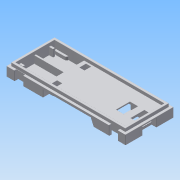
# Autodesk Inventor part: D2MG основание
Saved by Autodesk Inventor 2015 SP1 (Build 190203100, 203)
## iProperties
Created: 2017-11-06
Part Number: D2MG основание
Material: Типовые
Document SubType Name: Modeling
Designer: Влад
Density: 1 g/cm^3
Appearance: Белый пластик
Author: Влад
Autodesk Inventor part; units mm, degrees
ref_plane "YZ Plane" through (0, 0, 0) normal (1, 0, 0) x (0, 1, 0)
sketch "Эскиз1" plane through (0, 0, 0) normal (0, 0, 1) x (1, 0, 0)
  line L0 (-45.1, 18.15) -> (45.1, 18.15)
  line L1 (45.1, 18.15) -> (45.1, -18.15)
  line L2 (45.1, -18.15) -> (-45.1, -18.15)
  line L3 (-45.1, -18.15) -> (-45.1, 18.15)
  line L4 (-45.1, 18.15) -> (45.1, -18.15) construction
  line L5 (45.1, 18.15) -> (-45.1, -18.15) construction
  point P0 (0, 0)
  point P1 (0, 0)
  dimension "d0" = 90.2
  dimension "d1" = 36.3
  constraints: 12 end point, 2 parallel, 1 coincident, 1 horizontal, 1 midpoint, 1 perpendicular
  measures "d0" distance of L1.end L2.end
  measures "d1" distance of L0.end L1.end
extrude "Выдавливание1" add sketch "Эскиз1" along normal blind 2
sketch "Эскиз2" plane through (0, 0, 2) normal (0, 0, 1) x (1, 0, 0)
  line L0 (-43.25, 16.45) -> (43.25, 16.45)
  line L1 (43.25, 16.45) -> (43.25, -16.45)
  line L2 (43.25, -16.45) -> (-43.25, -16.45)
  line L3 (-43.25, -16.45) -> (-43.25, 16.45)
  line L4 (45.1, -18.15) -> (45.1, 18.15) projected
  line L5 (-45.1, 18.15) -> (-45.1, -18.15) projected
  line L6 (45.1, 18.15) -> (-45.1, 18.15) projected
  line L7 (-45.1, -18.15) -> (45.1, -18.15) projected
  line L8 (-41.55, 14.75) -> (41.55, 14.75)
  line L9 (41.55, 14.75) -> (41.55, -14.75)
  line L10 (41.55, -14.75) -> (-41.55, -14.75)
  line L11 (-41.55, -14.75) -> (-41.55, 14.75)
  point P0 (0, 0)
  dimension "d102" = 14.15
  dimension "d4" = 1.85
  dimension "d5" = 1.85
  dimension "d6" = 1.7
  dimension "d7" = 1.7
  dimension "d8" = 1.7
  dimension "d9" = 1.7
  dimension "d10" = 1.7
  dimension "d11" = 1.7
  constraints: 16 end point, 4 parallel, 2 horizontal, 2 perpendicular
  measures "d4" distance between parallel lines of L4 L1
  measures "d5" distance between parallel lines of L5 L3
  measures "d6" distance between parallel lines of L6 L0
  measures "d7" distance between parallel lines of L7 L2
  measures "d8" distance between parallel lines of L0 L8
  measures "d9" distance between parallel lines of L2 L10
  measures "d10" distance between parallel lines of L1 L9
  measures "d11" distance between parallel lines of L3 L11
extrude "Выдавливание2" add sketch "Эскиз2" along normal blind 2.4 contours L0 L1 L2 L3
sketch "Эскиз3" plane through (0, 0, 0) normal (0, 0, -1) x (-1, 0, 0)
  line L0 (7.1, -5.25) -> (-45.1, -5.25)
  line L1 (-45.1, -5.25) -> (-45.1, 5.25)
  line L2 (-45.1, 5.25) -> (7.1, 5.25)
  line L3 (7.1, 5.25) -> (7.1, -5.25)
  line L4 (45.1, -18.15) -> (45.1, 18.15) projected
  line L5 (-45.1, 18.15) -> (-45.1, -18.15) projected
  line L6 (45.1, 18.15) -> (-45.1, 18.15) projected
  line L7 (-45.1, -18.15) -> (45.1, -18.15) projected
  point P0 (0, 0)
  point P1 (-45.1, 0)
  dimension "d14" = 10.5
  dimension "d15" = 38
  dimension "d66" = 12.9
  dimension "d67" = 12.9
  constraints: 8 end point, 2 midpoint, 2 parallel, 1 horizontal, 1 perpendicular
  measures "d14" distance of L0.end L1.end
  measures "d15" distance between parallel lines of L4 L3
  measures "d66" distance between parallel lines of L6 L2
  measures "d67" distance between parallel lines of L7 L0
extrude "Выдавливание3" cut sketch "Эскиз3" against normal blind 1.1 contours L0 L1 L2 L3
sketch "Эскиз4" plane through (0, 0, 0) normal (0, 0, -1) x (-1, 0, 0)
  line L0 (-45.1, 18.15) -> (45.1, 18.15) projected
  line L1 (45.1, -18.15) -> (17.4, -18.15)
  line L2 (17.4, -18.15) -> (17.4, 18.15)
  line L3 (17.4, 18.15) -> (45.1, 18.15)
  line L4 (45.1, 18.15) -> (45.1, -18.15)
  point P0 (0, 0)
  dimension "d18" = 27.7
  constraints: 8 end point, 2 parallel, 1 horizontal, 1 perpendicular, 1 point on line
  measures "d18" distance of L2.end L3.end
extrude "Выдавливание4" add sketch "Эскиз4" along normal blind 5.1
sketch "Эскиз5" plane through (0, 0, -5.1) normal (0, 0, -1) x (-1, 0, 0)
  line L0 (39.1, -18.15) -> (32.6, -18.15)
  line L1 (32.6, -18.15) -> (32.6, -16.65)
  line L2 (32.6, -16.65) -> (39.1, -16.65)
  line L3 (39.1, -16.65) -> (39.1, -18.15)
  line L4 (39.1, 16.65) -> (32.6, 16.65)
  line L5 (32.6, 16.65) -> (32.6, 18.15)
  line L6 (32.6, 18.15) -> (39.1, 18.15)
  line L7 (39.1, 18.15) -> (39.1, 16.65)
  line L8 (45.1, -18.15) -> (45.1, 18.15) projected
  line L9 (17.4, -18.15) -> (45.1, -18.15) projected
  line L10 (45.1, 18.15) -> (17.4, 18.15) projected
  point P0 (0, 0)
  point P1 (35.85, -18.15)
  point P2 (35.85, 18.15)
  dimension "d21" = 6.5
  dimension "d22" = 1.5
  dimension "d23" = 6.5
  dimension "d24" = 1.5
  dimension "d25" = 6
  dimension "d26" = 6
  constraints: 16 end point, 4 parallel, 3 point on line, 2 horizontal, 2 midpoint, 2 perpendicular
  measures "d21" distance of L1.end L2.end
  measures "d22" distance of L0.end L1.end
  measures "d23" distance of L5.end L6.end
  measures "d24" distance of L4.end L5.end
  measures "d25" distance between parallel lines of L8 L3
  measures "d26" distance between parallel lines of L8 L7
extrude "Выдавливание5" cut sketch "Эскиз5" against normal through all
sketch "Эскиз6" plane through (0, 0, -5.1) normal (0, 0, -1) x (-1, 0, 0)
  line L0 (39.1, -16.65) -> (32.6, -16.65)
  line L1 (32.6, -16.65) -> (32.6, -15.15)
  line L2 (32.6, -15.15) -> (39.1, -15.15)
  line L3 (39.1, -15.15) -> (39.1, -16.65)
  line L4 (39.1, 16.65) -> (32.6, 16.65)
  line L5 (32.6, 16.65) -> (32.6, 15.15)
  line L6 (32.6, 15.15) -> (39.1, 15.15)
  line L7 (39.1, 15.15) -> (39.1, 16.65)
  point P0 (0, 0)
  dimension "d29" = 1.5
  dimension "d30" = 1.5
  constraints: 16 end point, 4 parallel, 2 horizontal, 2 perpendicular, 1 point on line
  measures "d29" distance of L0.end L1.end
  measures "d30" distance of L5.end L4.end
extrude "Выдавливание6" cut sketch "Эскиз6" against normal blind 3
sketch "Эскиз8" plane through (45.1, 18.15, 2) normal (0, 1, 0) x (1, 0, 0)
  line L0 (-26.5, 2) -> (-24.3, 7.1)
  line L1 (0, 7.1) -> (0, 2)
  line L2 (0, 2) -> (-62.5, 2) projected
  line L3 (-62.5, 2) -> (-62.5, 7.1) projected
  line L4 (-6, 7.1) -> (-6, 2)
  line L5 (-12.5, 2) -> (-12.5, 7.1)
  line L6 (-24.3, 7.1) -> (-12.5, 7.1)
  line L7 (-6, 7.1) -> (0, 7.1)
  line L8 (0, 2) -> (-6, 2)
  line L9 (-12.5, 2) -> (-26.5, 2)
  dimension "d34" = 36
  dimension "d35" = 38.2
  dimension "d38" = 6
  dimension "d39" = 6.5
  constraints: 16 end point, 2 collinear, 2 horizontal, 2 perpendicular, 2 point on line, 1 parallel
  measures "d34" distance of L2.end L0.start
  measures "d35" distance from line of L3 L0.end
  measures "d38" distance between parallel lines of L1 L4
  measures "d39" distance between parallel lines of L4 L5
extrude "Выдавливание7" add sketch "Эскиз8" against normal blind 2
sketch "Эскиз9" plane through (0, 0, 2) normal (0, 0, 1) x (1, 0, 0)
  line L0 (32.6, 18.15) -> (39.1, 18.15)
  line L1 (39.1, 18.15) -> (39.1, 16.45)
  line L2 (39.1, 16.45) -> (32.6, 16.45)
  line L3 (32.6, 16.45) -> (32.6, 18.15)
  line L4 (45.1, 16.15) -> (45.1, 5.25) projected
  line L5 (32.6, 18.15) -> (39.1, 18.15) projected
  point P0 (0, 0)
  point P1 (35.85, 18.15)
  dimension "d42" = 6.5
  dimension "d43" = 1.7
  dimension "d44" = 6
  constraints: 8 end point, 2 midpoint, 2 parallel, 1 horizontal, 1 perpendicular
  measures "d42" distance of L1.end L2.end
  measures "d43" distance of L0.end L1.end
  measures "d44" distance between parallel lines of L4 L1
extrude "Выдавливание8" cut sketch "Эскиз9" against normal blind 2
sketch "Эскиз10" plane through (0, 0, 0) normal (0, 0, -1) x (-1, 0, 0)
  line L0 (-45.1, 5.25) -> (7.1, 5.25) projected
  line L1 (-45.1, -18.15) -> (-45.1, 18.15) projected
  line L2 (-25.6, 5.25) -> (-45.1, 5.25)
  line L3 (-45.1, 5.25) -> (-45.1, 16.45)
  line L4 (-45.1, 16.45) -> (-43.1, 16.45)
  line L5 (-25.6, 7.25) -> (-25.6, 5.25)
  line L6 (-25.6, 7.25) -> (-43.1, 7.25)
  line L7 (-43.1, 7.25) -> (-43.1, 16.45)
  point P0 (0, 0)
  dimension "d47" = 19.5
  dimension "d48" = 2
  constraints: 12 end point, 2 horizontal, 2 parallel, 2 point on line, 1 perpendicular, 1 vertical
  measures "d47" distance between parallel lines of L1 L5
  measures "d48" distance between parallel lines of L6 L0
extrude "Выдавливание9" add sketch "Эскиз10" along normal blind 5.1
sketch "Эскиз11" plane through (0, 0, 0) normal (0, 0, -1) x (-1, 0, 0)
  line L0 (-31.1, 14.95) -> (-40.6, 14.95)
  line L1 (-40.6, 14.95) -> (-40.6, 16.45)
  line L2 (-40.6, 16.45) -> (-31.1, 16.45)
  line L3 (-31.1, 16.45) -> (-31.1, 14.95)
  line L4 (-39.1, 18.15) -> (-39.1, 16.45) projected
  line L5 (-32.6, 16.45) -> (-32.6, 18.15) projected
  line L6 (-43.25, 16.45) -> (43.25, 16.45) projected
  point P0 (0, 0)
  point P1 (-35.85, 16.45)
  dimension "d53" = 1.5
  dimension "d54" = 1.5
  dimension "d55" = 1.5
  constraints: 8 end point, 2 parallel, 1 horizontal, 1 midpoint, 1 perpendicular, 1 point on line
  measures "d53" distance between parallel lines of L4 L1
  measures "d54" distance between parallel lines of L5 L3
  measures "d55" distance between parallel lines of L2 L0
extrude "Выдавливание10" add sketch "Эскиз11" along normal blind 2
fillet "Сопряжение1" radius 1.5 2 edges at (31.1, 14.95, -1) (40.6, 14.95, -1)
sketch "Эскиз12" plane through (0, 0, 0) normal (0, 0, -1) x (-1, 0, 0)
  ellipse E0 centre (-22.9, 13.95) end of major axis (-24.5, 13.95) minor radius 1.2
  line L0 (7.1, 5.25) -> (7.1, -5.25) projected
  line L1 (-32.6, 18.15) -> (32.6, 18.15) projected
  point P0 (0, 0)
  dimension "d60" = 1.6
  dimension "d61" = 1.2
  dimension "d62" = 30
  dimension "d63" = 4.2
  constraints: 2 other
  measures "d62" distance from line of L0 point (-22.9, 13.95)
  measures "d63" distance from line of point (-22.9, 13.95) L1
extrude "Выдавливание11" add sketch "Эскиз12" along normal blind 3
mirror "Зеркальное отражение1" about plane through (0, 0, 0) normal (0, 1, 0) of "Выдавливание7", "Выдавливание8", "Выдавливание9", "Выдавливание10", "Сопряжение1", "Выдавливание11"
sketch "Эскиз15" plane through (45.1, -18.15, -5.1) normal (0, 0, -1) x (-1, 0, 0)
  line L0 (0, 23.4) -> (52.2, 23.4) projected
  line L1 (19.5, 12.9) -> (14.5, 12.9)
  line L2 (14.5, 12.9) -> (14.5, 23.4)
  line L3 (14.5, 23.4) -> (19.5, 23.4)
  line L4 (19.5, 23.4) -> (19.5, 12.9)
  line L5 (52.2, 12.9) -> (0, 12.9) projected
  line L6 (8.7, 12.9) -> (3.7, 12.9)
  line L7 (3.7, 12.9) -> (3.7, 23.4)
  line L8 (3.7, 23.4) -> (8.7, 23.4)
  line L9 (8.7, 23.4) -> (8.7, 12.9)
  point P0 (45.1, 18.15)
  dimension "d68" = 5
  dimension "d69" = 5
  dimension "d70" = 5.8
  constraints: 16 end point, 4 parallel, 3 point on line, 2 horizontal, 2 perpendicular
  measures "d68" distance of L2.end L3.end
  measures "d69" distance of L7.end L8.end
  measures "d70" distance between parallel lines of L9 L2
extrude "Выдавливание12" add sketch "Эскиз15" against normal blind 2 contours L0 L9 L5 L7 | L0 L4 L1 L2
sketch "Эскиз16" plane through (0, 0, 2) normal (0, 0, 1) x (1, 0, 0)
  line L0 (-7.1, -5.25) -> (45.1, -5.25) projected
  line L1 (-7.1, 5.25) -> (-7.1, -5.25) projected
  line L2 (45.1, 5.25) -> (-7.1, 5.25) projected
  line L3 (45.1, -5.25) -> (45.1, 5.25) projected
  line L4 (-7.1, -5.25) -> (45.1, -5.25) projected
  line L5 (36.1, 5.25) -> (42.1, 5.25)
  line L6 (42.1, 5.25) -> (42.1, -5.25)
  line L7 (42.1, -5.25) -> (36.1, -5.25)
  line L8 (36.1, -5.25) -> (36.1, 5.25)
  line L9 (45.1, 5.25) -> (-7.1, 5.25) projected
  line L10 (31.1, 5.25) -> (25.1, 5.25)
  line L11 (25.1, 5.25) -> (25.1, -5.25)
  line L12 (25.1, -5.25) -> (31.1, -5.25)
  line L13 (31.1, -5.25) -> (31.1, 5.25)
  point P0 (0, 0)
  dimension "d73" = 6
  dimension "d74" = 6
  dimension "d75" = 5
  dimension "d76" = 3
  constraints: 16 end point, 4 parallel, 4 point on line, 2 horizontal, 2 perpendicular
  measures "d73" distance of L6.end L7.end
  measures "d74" distance of L12.end L11.end
  measures "d75" distance between parallel lines of L8 L13
  measures "d76" distance between parallel lines of L3 L6
extrude "Выдавливание13" cut sketch "Эскиз16" against normal blind 2 contours L11 L2 L13 L0 | L8 L2 L6 L0
ref_plane "РабПлоскость1" through (-17.4, 13.35, 0) normal (0, 1, 0) x (1, 0, 0)
sketch "Эскиз17" plane through (-17.4, 13.35, 0) normal (0, 1, 0) x (1, 0, 0)
  line L0 (0, 5.1) -> (3, 5.1)
  line L1 (3, 5.1) -> (3, 3.4)
  line L2 (3, 3.4) -> (1, 2.1002)
  line L3 (1, 2.1002) -> (1, 0)
  line L4 (1, 0) -> (0, 0)
  line L5 (0, 0) -> (36, 0) projected
  line L6 (0, 0) -> (0, 5.1)
  point P0 (17.4, 0)
  dimension "d80" = 3
  dimension "d81" = 1.7
  dimension "d82" = 1
  constraints: 12 end point, 2 perpendicular, 1 collinear, 1 horizontal, 1 parallel
  measures "d80" distance of L0.start L0.end
  measures "d81" distance of L0.end L1.end
  measures "d82" distance of L3.end L4.end
extrude "Выдавливание14" add sketch "Эскиз17" against normal blind 4.8
ref_plane "РабПлоскость2" through (-17.4, 11.95, 0) normal (0, 1, 0) x (1, 0, 0)
sketch "Эскиз18" plane through (-17.4, 11.95, 0) normal (0, 1, 0) x (1, 0, 0)
  line L0 (3, 3.4) -> (3, 2.4328)
  line L1 (3, 2.4328) -> (1, 1.7474)
  line L2 (1, 2.1002) -> (1, 0) projected
  line L3 (1, 1.7474) -> (1, 2.1002)
  line L4 (3, 3.4) -> (1, 2.1002)
  point P0 (17.4, 0)
  constraints: 8 end point, 1 collinear, 1 point on line, 1 vertical
extrude "Выдавливание15" add sketch "Эскиз18" against normal blind 2
sketch "Эскиз19" plane through (0, 0, 0) normal (0, 0, -1) x (-1, 0, 0)
  line L0 (16.4, 8.45) -> (12.6, 8.45)
  line L1 (12.6, 8.45) -> (12.6, 13.45)
  line L2 (12.6, 13.45) -> (16.4, 13.45)
  line L3 (16.4, 13.45) -> (16.4, 8.45)
  line L4 (16.4, 8.55) -> (16.4, 13.35) projected
  line L5 (17.4, 18.15) -> (-18.6, 18.15) projected
  point P0 (0, 0)
  point P1 (16.4, 10.95)
  dimension "d88" = 3.8
  dimension "d89" = 5
  dimension "d90" = 4.7
  constraints: 8 end point, 2 midpoint, 2 parallel, 1 horizontal, 1 perpendicular
  measures "d88" distance between parallel lines of L4 L1
  measures "d89" distance between parallel lines of L2 L0
  measures "d90" distance between parallel lines of L5 L2
extrude "Выдавливание16" cut sketch "Эскиз19" against normal blind 2.5
mirror "Зеркальное отражение3" about plane through (0, 0, 0) normal (0, 1, 0) of "Выдавливание14", "Выдавливание15", "Выдавливание16"
sketch "Эскиз20" plane through (0, 0, 4.4) normal (0, 0, 1) x (1, 0, 0)
  line L0 (-41.55, 14.75) -> (-19.35, 14.75)
  line L1 (-19.35, 14.75) -> (-19.35, -14.75)
  line L2 (-19.35, -14.75) -> (-41.55, -14.75)
  line L3 (-41.55, -14.75) -> (-41.55, 14.75)
  line L4 (-41.55, -14.75) -> (41.55, -14.75) projected
  point P0 (0, 0)
  point P1 (-30.45, -14.75)
  dimension "d93" = 22.2
  dimension "d94" = 29.5
  constraints: 8 end point, 2 parallel, 1 horizontal, 1 midpoint, 1 perpendicular, 1 point on line
  measures "d93" distance of L1.end L2.end
  measures "d94" distance between parallel lines of L2 L0
extrude "Выдавливание17" cut sketch "Эскиз20" against normal blind 8
sketch "Эскиз21" plane through (0, 0, -3.6) normal (0, 0, 1) x (1, 0, 0)
  line L0 (-41.55, 14.75) -> (-19.35, 14.75) projected
  line L1 (-41.55, -14.75) -> (-41.55, 14.75) projected
  line L2 (-19.35, -14.75) -> (-41.55, -14.75) projected
  line L3 (-19.35, 14.75) -> (-19.35, -14.75) projected
  line L4 (-41.55, 0.6) -> (-19.35, 0.6)
  line L5 (-19.35, -0.6) -> (-41.55, -0.6)
  line L6 (-41.55, 12.1) -> (-38.55, 12.1)
  line L7 (-38.55, 12.1) -> (-38.55, 10.6)
  line L8 (-38.55, 10.6) -> (-41.55, 10.6)
  line L9 (-41.55, 10.6) -> (-41.55, 12.1)
  line L10 (-41.55, -10.6) -> (-38.55, -10.6)
  line L11 (-38.55, -10.6) -> (-38.55, -12.1)
  line L12 (-38.55, -12.1) -> (-41.55, -12.1)
  line L13 (-41.55, -12.1) -> (-41.55, -10.6)
  point P0 (0, 0)
  dimension "d101" = 14.15
  dimension "d102" = 14.15
  dimension "d103" = 1.2
  dimension "d106" = 3
  dimension "d107" = 1.5
  dimension "d108" = 10
  dimension "d109" = 3
  dimension "d110" = 1.5
  dimension "d111" = 10
  constraints: 20 end point, 6 point on line, 5 parallel, 3 horizontal, 2 perpendicular
  measures "d101" distance between parallel lines of L0 L4
  measures "d102" distance between parallel lines of L2 L5
  measures "d103" distance between parallel lines of L5 L4
  measures "d106" distance of L7.end L8.end
  measures "d107" distance of L6.end L7.end
  measures "d108" distance between parallel lines of L4 L8
  measures "d109" distance of L11.end L12.end
  measures "d110" distance of L10.end L11.end
  measures "d111" distance between parallel lines of L5 L10
extrude "Выдавливание19" add sketch "Эскиз21" along normal blind 5.5 contours L6 L7 L8 L1 | L3 L5 L1 L4 | L10 L11 L12 L1
sketch "Эскиз22" plane through (0, 0, -3.6) normal (0, 0, 1) x (1, 0, 0)
  line L0 (-40.6, -13.25) -> (-31.1, -13.25)
  line L1 (-31.1, -13.25) -> (-31.1, -14.75)
  line L2 (-31.1, -14.75) -> (-40.6, -14.75)
  line L3 (-40.6, -14.75) -> (-40.6, -13.25)
  line L4 (-39.1, -15.15) -> (-39.1, -18.15) projected
  line L5 (-32.6, -16.65) -> (-32.6, -18.15) projected
  line L6 (-32.6, -18.15) -> (-32.6, -15.15) projected
  line L7 (-19.35, -14.75) -> (-41.55, -14.75) projected
  point P0 (0, 0)
  point P1 (-35.85, -14.75)
  dimension "d114" = 1.5
  dimension "d115" = 1.5
  dimension "d117" = 1.5
  constraints: 8 end point, 2 parallel, 1 horizontal, 1 midpoint, 1 perpendicular, 1 point on line
  measures "d114" distance of L0.end L1.end
  measures "d115" distance between parallel lines of L4 L3
  measures "d117" distance between parallel lines of L6 L1
extrude "Выдавливание20" add sketch "Эскиз22" along normal blind 2.5
fillet "Сопряжение2" radius 1.5 2 edges at (-31.1, -13.25, -2.35) (-40.6, -13.25, -2.35)
mirror "Зеркальное отражение4" about plane through (0, 0, 0) normal (0, 1, 0) of "Выдавливание20", "Сопряжение2"
fillet "Сопряжение3" radius 0.1 26 edges at (-38.55, 10.6, -0.85) (-38.55, 12.1, -0.85) (-38.55, 11.35, 1.9) (-40.05, 10.6, 1.9) (-40.05, 12.1, 1.9) (-38.55, -11.35, 1.9) (-40.05, -12.1, 1.9) (-38.55, -12.1, -0.85) (-38.55, -10.6, -0.85) (-40.05, -10.6, 1.9) (-40.1607, 13.6893, -1.1) (-40.6, 14.7499, -1.1) (-31.5393, 13.6893, -1.1) (-31.1, 14.7499, -1.1) (-35.85, 13.25, -1.1) (-40.6, -14.7499, -1.1) (-40.1607, -13.6893, -1.1) (-31.5393, -13.6893, -1.1) (-31.1, -14.7499, -1.1) (-35.85, -13.25, -1.1) (31.621, -15.2881, -2) (40.079, -15.2881, -2) (35.85, -14.95, -2) (31.621, 15.2881, -2) (40.079, 15.2881, -2) (35.85, 14.95, -2)
fillet "Сопряжение4" radius 0.2 22 edges at (-19.35, 0, 2) (0, -18.15, 2) (-42.1, -18.15, 2) (-45.1, 0, 2) (-42.1, 18.15, 2) (-39.1, 17.4, 2) (-32.6, 17.4, 2) (0, 18.15, 2) (32.6, 17.3, 2) (39.1, 17.3, 2) (42.1, 18.15, 2) (45.1, 0, 2) (42.1, -18.15, 2) (39.1, -17.3, 2) (32.6, -17.3, 2) (43.25, 0, 4.4) (0, 16.45, 4.4) (43.25, 16.45, 3.2) (-43.25, 16.45, 3.2) (-43.25, 0, 4.4) (-43.25, -16.45, 3.2) (0, -16.45, 4.4)
fillet "Сопряжение5" radius 0.3 37 edges at (-45.1, 0, -5.1) (-42.1, 18.15, -5.1) (-45.0414, 18.0914, 1.9414) (-45.1, 18.15, -1.65) (-32.5414, 18.0914, 1.9414) (-32.6, 18.15, -1.65) (-39.1586, 18.0914, 1.9414) (-39.1, 18.15, -1.65) (-17.4, 18.15, -2.55) (-25, 18.15, -5.1) (-17.4, 15.75, -5.1) (-17.4, 0, -5.1) (-14.4, 10.95, -5.1) (-15.9, 13.35, -5.1) (-14.4, 13.35, -4.25) (-17.4, -15.75, -5.1) (-15.9, -13.35, -5.1) (-14.4, -10.95, -5.1) (-15.9, -8.55, -5.1) (-14.4, -8.55, -4.25) (-14.4, -13.35, -4.25) (-14.4, 8.55, -4.25) (0.6, 18.15, 0) (19.7, 18.15, -2.55) (26.7, 18.15, -5.1) (32.5414, 18.0914, 1.9414) (32.6, 18.15, -1.65) (42.1, 18.15, -5.1) (39.1586, 18.0914, 1.9414) (39.1, 18.15, -1.65) (45.0414, 18.0914, 1.9414) (45.1, 18.15, -1.65) (45.1, 11.7, -5.1) (45.1, 5.25, -2) (45.1, -5.25, -2) (45.0414, -18.0914, 1.9414) (45.1, -18.15, -1.65)
fillet "Сопряжение6" radius 0.3 13 edges at (-45.0121, -18.15, -5.0121) (-41.95, -18.15, -5.1) (-45.0414, -18.0914, 1.9414) (-45.1, -18.15, -1.5) (-17.4879, -18.15, -5.0121) (-17.4, -18.15, -2.4) (-25.15, -18.15, -5.1) (-32.6, -18.0914, 1.9414) (-32.6, -17.3, 2) (-32.6, -18.15, -1.65) (-39.1, -18.0914, 1.9414) (-39.1, -17.3, 2) (-39.1, -18.15, -1.65)
fillet "Сопряжение7" radius 0.3 12 edges at (0.45, -18.15, 0) (19.7, -18.15, -2.55) (26.7, -18.15, -5.1) (32.5414, -18.0914, 1.9414) (32.6, -18.15, -1.65) (39.1586, -18.0914, 1.9414) (39.1, -18.15, -1.65) (45.0121, -18.0621, -5.1) (45.1, -11.7, -5.1) (45.0121, -5.3379, -5.1) (43.1, -5.25, -5.1) (41.95, -18.15, -5.1)
fillet "Сопряжение8" radius 0.2 11 edges at (25.6, 0, -5.1) (41.4, -0.15, -5.1) (45.0121, 5.3379, -5.0121) (43.1, 5.25, -5.1) (34.35, -7.25, -5.1) (34.35, 7.25, -5.1) (25.6, -7.25, -2.55) (25.6, 7.25, -2.55) (9.25, 5.25, 0) (-7.1, 0, 0) (9.25, -5.25, 0)
fillet "Сопряжение9" radius 0.2 11 edges at (0, -14.75, 4.4) (-41.55, 0, 4.4) (0, 14.75, 4.4) (41.55, 0, 4.4) (25.1, 0, 2) (28.1, -5.25, 2) (31.1, 0, 2) (28.1, 5.25, 2) (38.825, 5.25, 2) (36.1, 0, 2) (38.825, -5.25, 2)
fillet "Сопряжение10" radius 0.2 1 edges at (41.55, 0, 2)
fillet "Сопряжение11" radius 0.1 8 edges at (-14.5, -13.45, 2) (-12.6, -10.95, 2) (-14.5, -8.45, 2) (-16.4, -10.95, 2) (-14.5, 8.45, 2) (-12.6, 10.95, 2) (-16.4, 10.95, 2) (-14.5, 13.45, 2)
fillet "Сопряжение12" radius 0.2 2 edges at (21.3, -13.95, -3) (21.3, 13.95, -3)
fillet "Сопряжение13" radius 0.1 6 edges at (-14.5, 8.45, 0) (-12.6, 10.95, 0) (-14.5, 13.45, 0) (-14.5, -13.45, 0) (-12.6, -10.95, 0) (-14.5, -8.45, 0)
ref_plane "РабПлоскость4" through (-17.4, -11.95, 0) normal (0, 1, 0) x (1, 0, 0)
